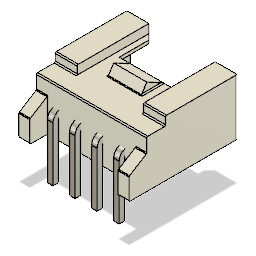
GroveConnector_110990037 (Autodesk Fusion 360 design; units mm, degrees)
Autodesk Fusion 360 part; units mm, degrees
sketch "Sketch1" plane through (0, 0, 0) normal (0, 1, 0) x (1, 0, 0)
  line L0 (2.25, 0) -> (-7.75, 0)
  line L1 (-7.75, 0) -> (-7.75, 8.2)
  line L2 (-7.75, 8.2) -> (2.25, 8.2)
  line L3 (2.25, 8.2) -> (2.25, 0)
  dimension "d1" = 2.25
  dimension "d2" = 7.75
  dimension "d3" = 8.2
  measures "d1" distance of origin
  measures "d2" distance of origin
extrude "Extrude1" add sketch "Sketch1" along normal blind 5.1 makes body 1
sketch "Sketch2" plane through (2.25, 0, 0) normal (1, 0, 0) x (0, 0, -1)
  line L0 (0, 0) -> (8.2, 0)
  line L1 (8.2, 0) -> (8.2, 5.1)
  line L2 (8.2, 5.1) -> (0, 5.1)
  line L3 (0, 5.1) -> (0, 0)
  line L4 (1.7, 5.1) -> (0, 5.1)
  line L5 (0, 5.1) -> (0, 4.3)
  line L6 (0, 4.3) -> (1.7, 4.3)
  line L7 (1.7, 4.3) -> (1.7, 5.1)
  dimension "d6" = 6.5
  dimension "d7" = 0.8
  measures "d6" distance of L1
extrude "Extrude2" cut sketch "Sketch2" against normal through all contours L2 L3 L4 L5 L6 L7 bodies 1
ref_plane "WorkPlane1" through (-2.75, 2.55, -4.1) normal (1, 0, 0) x (0, 0, -1)
sketch "Sketch3" plane through (2.25, 0, 0) normal (1, 0, 0) x (0, 0, -1)
  line L0 (1.7, 4.3) -> (0, 4.3)
  line L1 (0, 4.3) -> (0, 0)
  line L2 (0, 0) -> (8.2, 0)
  line L3 (8.2, 0) -> (8.2, 5.1)
  line L4 (8.2, 5.1) -> (1.7, 5.1)
  line L5 (1.7, 5.1) -> (1.7, 4.3)
  line L6 (0, 0) -> (-1.6, 0)
  line L7 (-1.6, 0) -> (-1.6, 2)
  line L8 (-1.6, 2) -> (0, 3)
  dimension "d9" = 1.6
  dimension "d10" = 2
  dimension "d11" = 1
  measures "d9" distance of L1.end
extrude "Extrude3" add sketch "Sketch3" against normal blind 1 separate body contours L1 L6 L7 L8 makes body 2
mirror "Mirror1" about plane through (-2.75, 2.55, -4.1) normal (1, 0, 0) of bodies 2 makes body 3
sketch "Sketch4" plane through (0, 0, -8.2) normal (0, 0, -1) x (-1, 0, 0)
  line L0 (-2.25, 0) -> (7.75, 0)
  line L1 (7.75, 0) -> (7.75, 5.1)
  line L2 (7.75, 5.1) -> (-2.25, 5.1)
  line L3 (-2.25, 5.1) -> (-2.25, 0)
  line L4 (-0.25, 5.1) -> (5.75, 5.1)
  line L5 (5.75, 5.1) -> (5.75, 4.3)
  line L6 (5.75, 4.3) -> (-0.25, 4.3)
  line L7 (-0.25, 4.3) -> (-0.25, 5.1)
  line L8 (-2.25, 4.3) -> (7.75, 4.3) construction
  line L9 (2.75, 5.61) -> (2.75, -0.51) construction
  dimension "d15" = 2
  measures "d15" distance of L3 L7
extrude "Extrude4" cut sketch "Sketch4" against normal through all contours L2 L4 L5 L6 L7 bodies 1
shell "Shell1" thickness 0.5 removed faces 1 at (-3.75, 1.4333, -8.2) on bodies 1
sketch "Sketch5" plane through (0, 0, 0) normal (0, -1, 0) x (1, 0, 0)
  line L0 (-7.75, -8.2) -> (2.25, -8.2)
  line L1 (2.25, -8.2) -> (2.25, 0)
  line L2 (2.25, 0) -> (-7.75, 0)
  line L3 (-7.75, 0) -> (-7.75, -8.2)
  line L4 (-6.25, -8.2) -> (0.75, -8.2)
  line L5 (0.75, -8.2) -> (0.75, -7.2)
  line L6 (0.75, -7.2) -> (-6.25, -7.2)
  line L7 (-6.25, -7.2) -> (-6.25, -8.2)
  line L8 (-6.25, -8.2) -> (-6.25, -2.2)
  line L9 (0.75, -8.2) -> (0.75, -2.2)
  dimension "d18" = 1
extrude "Extrude5" cut sketch "Sketch5" against normal blind 0.5 contours L0 L4 L5 L6 L7 L8 L9 bodies 1
sketch "Sketch6" plane through (0, 4.3, 0) normal (0, 1, 0) x (-1, 0, 0)
  line L0 (7.75, -1.7) -> (7.75, 0)
  line L1 (7.75, 0) -> (-2.25, 0)
  line L2 (-2.25, 0) -> (-2.25, -1.7)
  line L3 (-2.25, -1.7) -> (-0.25, -1.7)
  line L4 (-0.25, -1.7) -> (-0.25, -8.2)
  line L5 (-0.25, -8.2) -> (5.75, -8.2)
  line L6 (5.75, -8.2) -> (5.75, -1.7)
  line L7 (5.75, -1.7) -> (7.75, -1.7)
  line L8 (5.75, -8.2) -> (5.25, -7.7)
  line L9 (5.25, -7.7) -> (5.25, -5)
  line L10 (5.25, -5) -> (2.75, -5)
  line L11 (2.75, 0.82) -> (2.75, -9.02) construction
  line L12 (5.75, -8.2) -> (2.75, -8.2)
  line L13 (-0.25, -8.2) -> (0.25, -7.7)
  line L14 (0.25, -7.7) -> (0.25, -5)
  line L15 (0.25, -5) -> (2.75, -5)
  line L16 (-0.25, -8.2) -> (2.75, -8.2)
  dimension "d21" = 45
  dimension "d22" = 0.5
  dimension "d23" = 3.2
  measures "d21" angle of L8 L12
  measures "d22" distance of L6 L9
  measures "d23" distance of L10 L12
extrude "Extrude6" cut sketch "Sketch6" against normal blind 0.5 contours L5 L8 L9 L10 L12 L13 L14 L15 L16 bodies 1
sketch "Sketch7" plane through (0, 4.3, 0) normal (0, 1, 0) x (-1, 0, 0)
  line L0 (-0.25, -8.2) -> (0.25, -7.7)
  line L1 (0.25, -7.7) -> (0.25, -5)
  line L2 (0.25, -5) -> (5.25, -5)
  line L3 (5.25, -5) -> (5.25, -7.7)
  line L4 (5.25, -7.7) -> (5.75, -8.2)
  line L5 (5.75, -8.2) -> (5.75, -1.7)
  line L6 (5.75, -1.7) -> (7.75, -1.7)
  line L7 (7.75, -1.7) -> (7.75, 0)
  line L8 (7.75, 0) -> (-2.25, 0)
  line L9 (-2.25, 0) -> (-2.25, -1.7)
  line L10 (-2.25, -1.7) -> (-0.25, -1.7)
  line L11 (-0.25, -1.7) -> (-0.25, -8.2)
  line L12 (4.25, -5) -> (1.25, -5)
  line L13 (1.25, -5) -> (1.25, -3)
  line L14 (1.25, -3) -> (4.25, -3)
  line L15 (4.25, -3) -> (4.25, -5)
  line L16 (2.75, 0.82) -> (2.75, -9.02) construction
  dimension "d26" = 2
  dimension "d27" = 3
extrude "Extrude7" add sketch "Sketch7" along normal blind 0.8 separate body contours L2 L12 L13 L14 L15 makes body 4
sketch "Sketch8" plane through (-1.25, 0, 0) normal (1, 0, 0) x (0, 0, -1)
  line L0 (5, 4.3) -> (5, 5.1)
  line L1 (5, 5.1) -> (3, 5.1)
  line L2 (3, 5.1) -> (3, 4.3)
  line L3 (5, 4.3) -> (3.5, 5.1)
  line L4 (3, 4.3) -> (3.5, 5.1)
  line L5 (5, 4.3) -> (3, 4.3)
  line L6 (3, 4.3) -> (5, 4.3)
  dimension "d30" = 0.5
extrude "Extrude8" cut sketch "Sketch8" against normal blind 3 contours L3 L4 L5 L6 keep common part bodies 4
sketch "Sketch9" plane through (0, 0, 0) normal (1, 0, 0) x (0, 0, -1)
  line L0 (-0.25, -3.4) -> (-0.25, 1.65)
  line L1 (0.25, 2.15) -> (6.75, 2.15)
  arc A0 (0.25, 2.15) -> (-0.25, 1.65) centre (0.25, 1.65) ccw
  dimension "d33" = 7
  dimension "d34" = 2.15
  dimension "d35" = 0.25
  dimension "d36" = 3.4
  dimension "d37" = 0.5
  measures "d34" distance of origin
  measures "d35" distance of origin
  measures "d36" distance of origin
  measures "d37" radius of A0
ref_plane "WorkPlane2" through (0, -3.4, 0.25) normal (0, 1, 0) x (-1, 0, 0)
sketch "Sketch10" plane through (0, -3.4, 0.25) normal (0, 1, 0) x (1, 0, 0)
  line L0 (0.25, 0.25) -> (-0.25, 0.25)
  line L1 (-0.25, 0.25) -> (-0.25, -0.25)
  line L2 (-0.25, -0.25) -> (0.25, -0.25)
  line L3 (0.25, -0.25) -> (0.25, 0.25)
  line L4 (0.25, 0.25) -> (-0.25, -0.25) construction
  line L5 (-0.25, 0.25) -> (0.25, -0.25) construction
  dimension "d46" = 0.5
  dimension "d47" = 0.5
sweep "Sweep2" add profiles "Sketch10" path "Sketch9" along L0 A0 L1 section 1 separate body makes body 5
chamfer "Chamfer1" distance 0.1 angle 45 4 edges at (0, -3.4, 0) (-0.25, -3.4, 0.25) (0, -3.4, 0.5) (0.25, -3.4, 0.25) on bodies 5
chamfer "Chamfer2" distance 0.1 angle 45 4 edges at (0, 2.4, -6.75) (0.25, 2.15, -6.75) (0, 1.9, -6.75) (-0.25, 2.15, -6.75) on bodies 5
pattern_linear "R-Pattern1" count 4 spacing 2 along (-1, 0, 0) of bodies 5 makes body 6 at (-1.75, 2.0667, -4.5167) makes body 7 at (-3.75, 2.0667, -4.5167) makes body 8 at (-5.75, 2.0667, -4.5167)
combine "Combine1" operation add target body 1 tool bodies 4 3 2
fillet "Fillet1" radius 0.1 13 edges at (1.25, 5.1, -1.7) (-6.75, 5.1, -1.7) (-6.75, 4.3, -1.7) (1.25, 4.3, -1.7) (-2.75, 4.3, 0) (1.75, 3, 0) (-7.25, 3, 0) (-7.25, 2, 1.6) (1.75, 2, 1.6) (1.75, 0, 1.6) (-7.25, 0, 1.6) (2.25, 2.55, -8.2) (-7.75, 2.55, -8.2) on bodies 1
fillet "Fillet2" radius 0.1 3 edges at (-4.25, 4.3, -4) (-2.75, 4.3, -3) (-1.25, 4.3, -4) on bodies 1
chamfer "Chamfer3" distance 0.2 angle 45 18 edges at (-6.75, 4.6, -8.2) (-7.25, 2.55, -8.2) (-6.75, 0.5, -8.2) (-6.25, 0.5, -7.7) (-2.75, 0.5, -7.2) (0.75, 0.5, -7.7) (1.25, 0.5, -8.2) (1.75, 2.55, -8.2) (1.25, 4.6, -8.2) (0.75, 4.2, -8.2) (0.5, 3.8, -8.2) (0, 3.8, -7.95) (-0.25, 3.8, -6.35) (-2.75, 3.8, -5) (-5.25, 3.8, -6.35) (-5.5, 3.8, -7.95) (-6, 3.8, -8.2) (-6.25, 4.2, -8.2) on bodies 1
named bodies: "Connector"
